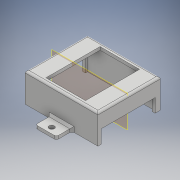
# Autodesk Inventor part: Eletronica - ProtecaoRele
Saved by Autodesk Inventor 2017 (Build 210142000, 142)
## iProperties
Created: 2020-10-18
Part Number: Eletronica - ProtecaoRele
Material: Generic
Document SubType Name: Modeling
Designer: ale
Density: 1 g/cm^3
Appearance: Default
Author: ale
Autodesk Inventor part; units mm, degrees
ref_plane "YZ Plane" through (0, 0, 0) normal (1, 0, 0) x (0, 1, 0)
ref_plane "XZ Plane" through (0, 0, 0) normal (0, 1, 0) x (-1, 0, 0)
ref_plane "XY Plane" through (0, 0, 0) normal (0, 0, 1) x (1, 0, 0)
sketch "Sketch1" plane through (0, 0, 0) normal (0, 0, 1) x (1, 0, 0)
  line L0 (-32, 27) -> (32, 27)
  line L1 (32, 27) -> (32, -27)
  line L2 (32, -27) -> (-32, -27)
  line L3 (-32, -27) -> (-32, 27)
  line L4 (-32, 27) -> (32, -27) construction
  line L5 (32, 27) -> (-32, -27) construction
  line L6 (35, 30) -> (-35, 30)
  line L7 (-35, 30) -> (-35, -30)
  line L8 (-35, -30) -> (35, -30)
  line L9 (35, -30) -> (35, 30)
  point P0 (0, 0)
  dimension "d0" = 64
  dimension "d1" = 54
  dimension "d2" = 3
  constraints: 20 end point, 4 parallel, 2 midpoint, 2 perpendicular, 1 horizontal, 3 other
  measures "d0" distance of L1.end L2.end
  measures "d1" distance of L0.end L1.end
  measures "d2" distance between parallel lines of L0 L6
extrude "Extrusion1" add sketch "Sketch1" along normal blind 25
sketch "Sketch2" plane through (0, 0, 25) normal (0, 0, 1) x (1, 0, 0)
  line L0 (35, 30) -> (-35, 30) projected
  line L1 (35, -30) -> (35, 30) projected
  line L2 (-35, 30) -> (35, 30)
  line L3 (35, 30) -> (35, -30)
  line L4 (35, -30) -> (-35, -30)
  line L5 (-35, -30) -> (-35, 30)
  point P0 (0, 0)
  constraints: 8 end point, 2 parallel, 1 horizontal, 1 perpendicular
extrude "Extrusion2" add sketch "Sketch2" along normal blind 3
sketch "Sketch3" plane through (35, -30, 0) normal (1, 0, 0) x (0, 0, -1)
  line L0 (0, 3) -> (-13, 3)
  line L1 (-13, 3) -> (-13, 55)
  line L2 (-13, 55) -> (0, 55)
  line L3 (0, 55) -> (0, 3)
  line L4 (0, 3) -> (-13, 55) construction
  line L5 (-13, 3) -> (0, 55) construction
  line L6 (0, 0) -> (0, 60) projected
  point P0 (0, 30)
  point P1 (-6.5, 29)
  dimension "d7" = 13
  dimension "d8" = 52
  dimension "d9" = 6.5
  constraints: 12 end point, 2 midpoint, 2 parallel, 1 horizontal, 1 perpendicular
  measures "d7" distance of L1.end L2.end
  measures "d8" distance of L0.end L1.end
  measures "d9" distance from line of L6 point (-6.5, 29)
extrude "Extrusion3" cut sketch "Sketch3" against normal through all
sketch "Sketch4" plane through (-35, -30, 0) normal (0, -1, 0) x (1, 0, 0)
  point P0 (35, 0)
sketch "Sketch5" plane through (0, 0, 0) normal (0, 0, -1) x (-1, 0, 0)
  line L0 (10, -30) -> (-10, -30)
  line L1 (-10, -30) -> (-10, -45)
  line L2 (-10, -45) -> (10, -45)
  line L3 (10, -45) -> (10, -30)
  line L4 (10, -30) -> (-10, -45) construction
  line L5 (-10, -30) -> (10, -45) construction
  line L6 (35, -27) -> (-35, -27) projected
  point P0 (0, 0)
  point P1 (0, -37.5)
  dimension "d12" = 20
  dimension "d13" = 15
  dimension "d14" = 10.5
  constraints: 12 end point, 2 midpoint, 2 parallel, 1 horizontal, 1 perpendicular
  measures "d12" distance of L2.end L1.end
  measures "d13" distance of L1.end L0.end
  measures "d14" distance from line of point (0, -37.5) L6
extrude "Extrusion4" add sketch "Sketch5" against normal blind 3
ref_plane "Work Plane1" through (-35, -1, 28) normal (0, -1, 0) x (1, 0, 0)
mirror "Mirror1" about plane through (-35, -1, 28) normal (0, -1, 0) of "Extrusion4"
chamfer "Chamfer1" distance 2 angle 45 6 edges at (10, -30, 1.5) (0, -30, 3) (-10, -30, 1.5) (10, 30, 1.5) (0, 30, 3) (-10, 30, 1.5)
fillet "Fillet1" radius 2 8 edges at (10, -45, 1.5) (-10, -45, 1.5) (-35, 0, 28) (0, -30, 28) (35, 0, 28) (0, 30, 28) (10, 43, 1.5) (-10, 43, 1.5)
sketch "Sketch7" plane through (0, 0, 28) normal (0, 0, 1) x (1, 0, 0)
  line L0 (-19, -26) -> (19, -26)
  line L1 (19, -26) -> (19, 26)
  line L2 (19, 26) -> (-19, 26)
  line L3 (-19, 26) -> (-19, -26)
  line L4 (-19, -26) -> (19, 26) construction
  line L5 (19, -26) -> (-19, 26) construction
  point P0 (0, 0)
  dimension "d25" = 38
  dimension "d26" = 52
  constraints: 12 end point, 2 midpoint, 2 parallel, 1 horizontal, 1 perpendicular
  measures "d25" distance of L2.end L1.end
  measures "d26" distance of L1.end L0.end
extrude "Extrusion6" cut sketch "Sketch7" against normal blind 3
sketch "Sketch8" plane through (-10, 32, 3) normal (0, 0, 1) x (1, 0, 0)
  line L0 (2, 11) -> (18, 11) projected
  line L1 (20, 9) -> (20, 0) projected
  point P0 (10, -32)
  point P1 (10, 5.5)
  dimension "d29" = 5.5
  dimension "d30" = 10
  measures "d29" distance from line of L0 point (10, 5.5)
  measures "d30" distance from line of point (10, 5.5) L1
hole "Hole1" at (0, 37.5, 3) direction (0, 0, -1) diameter 5 end through all
mirror "Mirror2" about plane through (-35, -1, 28) normal (0, -1, 0) of "Hole1"
body "Solid1"
